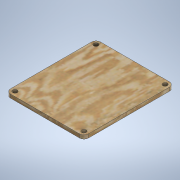
# Autodesk Inventor part: Tabletop
Saved by Autodesk Inventor 2020.2 (Build 242310000, 310)
## iProperties
Created: 2020-08-20
Part Number: Tabletop
Material: Generic
Document SubType Name: Modeling
Designer: JK
Density: 1 g/cm^3
Appearance: Plywood - Weathered
Author: JK
Autodesk Inventor part; units mm, degrees
ref_plane "YZ Plane" through (0, 0, 0) normal (1, 0, 0) x (0, 1, 0)
ref_plane "XZ Plane" through (0, 0, 0) normal (0, 1, 0) x (-1, 0, 0)
ref_plane "XY Plane" through (0, 0, 0) normal (0, 0, 1) x (1, 0, 0)
sketch "Sketch1" plane through (0, 0, 0) normal (0, 1, 0) x (-1, 0, 0)
  line L0 (-130, 150) -> (130, 150)
  line L1 (130, 150) -> (130, -150)
  line L2 (130, -150) -> (-130, -150)
  line L3 (-130, -150) -> (-130, 150)
  line L4 (-130, 150) -> (130, -150) construction
  line L5 (130, 150) -> (-130, -150) construction
  circle A0 centre (115, 135) radius 7.4
  circle A1 centre (-115, 135) radius 7.4
  circle A2 centre (115, -135) radius 7.4
  circle A3 centre (-115, -135) radius 7.4
  point P0 (0, 0)
  dimension "d0" = 260
  dimension "d1" = 300
  dimension "d2" = 14.8
  dimension "d3" = 15
  dimension "d4" = 15
  dimension "d5" = 15
  dimension "d6" = 15
  constraints: 12 end point, 4 centre point, 3 equal radius, 2 horizontal alignment, 2 midpoint, 2 parallel, 2 vertical alignment, 1 horizontal, 1 perpendicular
  measures "d0" distance between parallel lines of L1 L3
  measures "d1" distance of L0.end L1.end
  measures "d2" diameter of A0
  measures "d3" distance from line of L1 A0.centre
  measures "d4" distance from line of L0 A0.centre
  measures "d5" distance from line of A1.centre L3
  measures "d6" distance from line of L2 A2.centre
extrude "Extrusion1" add sketch "Sketch1" along normal blind 12
fillet "Fillet1" radius 15 4 edges at (130, 6, 150) (130, 6, -150) (-130, 6, 150) (-130, 6, -150)
body "Solid1"
